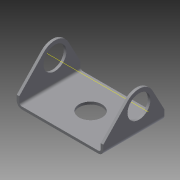
# Autodesk Inventor part: Bearing Mount 4 v1
Saved by Autodesk Inventor 2013 (Build 170138000, 138)
## iProperties
Created: 2013-01-18
Part Number: Bearing Mount 4 v1
Material: Generic
Document SubType Name: Sheet Metal
Designer: actoennies
Density: 1 g/cm^3
Flat Pattern Width: 7.62 cm
Flat Pattern Length: 19.8513 cm
Flat Pattern Area: 151.267 cm^2
Sheet Metal Rule: Default
Sheet Metal Width: 3.000 in
Sheet Metal Length: 7.815 in
Sheet Metal Area: 23.446 in^2
Mass: 35.0244 g
Surface Area: 244.107 cm^2
Volume: 35.0244 cm^3
Author: actoennies
Autodesk Inventor part; units mm, degrees
ref_plane "YZ Plane" through (0, 0, 0) normal (1, 0, 0) x (0, 1, 0)
ref_plane "XZ Plane" through (0, 0, 0) normal (0, 1, 0) x (-1, 0, 0)
ref_plane "XY Plane" through (0, 0, 0) normal (0, 0, 1) x (1, 0, 0)
sketch "Sketch1" plane through (0, 0, 0) normal (0, 1, 0) x (-1, 0, 0)
  line L0 (0, 0) -> (101.6, 0)
  line L1 (101.6, 0) -> (101.6, 76.2)
  line L2 (101.6, 76.2) -> (0, 76.2)
  line L3 (0, 76.2) -> (0, 0)
  dimension "d0" = 101.6
  dimension "d2" = 76.2
  measures "d0" distance of L1.end L2.end
  measures "d2" distance of L0.end L1.end
extrude "Plate1" add sketch "Sketch1" along normal blind 3.175
sketch "Sketch2" plane through (-101.6, 3.175, 76.2) normal (-1, 0, 0) x (0, -1, 0)
  line L0 (0, -76.2) -> (0, 0)
  line L1 (0, 0) -> (-47.625, 0)
  line L2 (-47.625, 0) -> (-47.625, -76.2)
  line L3 (-47.625, -76.2) -> (0, -76.2)
  constraints: 6 end point, 1 horizontal, 1 perpendicular, 1 vertical
edge flange "Flange1" height 50.8 angle 90 thickness 3.175 bend radius 3.175 thickness toward (-1, 0, 0) relief straight relief width 3.175 relief depth 1.5875 edges at (-101.6, 3.175, 38.1) wall of the first edge with corners at (-101.6, 3.175, 0) (-101.6, 3.175, 76.2) (-101.6, 50.8, 76.2) (-101.6, 50.8, 0)
bend "Bend1"
corner "Corner1"
sketch "Sketch3" plane through (0, 3.175, 0) normal (1, 0, 0) x (0, 1, 0)
  line L0 (0, 76.2) -> (0, 0)
  line L1 (0, 0) -> (47.625, 0)
  line L2 (47.625, 0) -> (47.625, 76.2)
  line L3 (47.625, 76.2) -> (0, 76.2)
  constraints: 6 end point, 1 horizontal, 1 perpendicular, 1 vertical
edge flange "Flange2" height 50.8 angle 90 thickness 3.175 bend radius 3.175 thickness toward (1, 0, 0) relief straight relief width 3.175 relief depth 1.5875 edges at (0, 3.175, 38.1) wall of the first edge with corners at (0, 3.175, 76.2) (0, 3.175, 0) (0, 50.8, 0) (0, 50.8, 76.2)
bend "Bend2"
corner "Corner2"
sketch "Sketch4" plane through (-101.6, 50.8, 76.2) normal (1, 0, 0) x (0, 0, -1)
  line L0 (76.2, 0) -> (0, 0) projected
  circle A0 centre (44.45, -19.05) radius 14.2875
  point P0 (76.2, -50.8)
  dimension "d24" = 28.575
  dimension "d25" = 19.05
  constraints: 1 centre point
  measures "d24" diameter of A0
  measures "d25" distance from line of L0 A0.centre
extrude "Cut1" cut sketch "Sketch4" against normal mid plane 5080
sketch "Sketch5" plane through (3.175, 50.8, 76.2) normal (1, 0, 0) x (0, 0, -1)
  circle A0 centre (44.45, -19.05) radius 14.2875 projected
  line L0 (0, -44.45) -> (76.2, -44.45) projected
  line L1 (76.2, 0) -> (76.2, -44.45) projected
  line L2 (0, 0) -> (76.2, 0) projected
  line L3 (0, -44.45) -> (0, 0) projected
  arc A1 (61.2588, -10.0853) -> (30.6552, -5.9121) centre (44.45, -19.05) ccw
  line L4 (0, -38.1) -> (30.6552, -5.9121)
  line L5 (61.2588, -10.0853) -> (76.2, -38.1)
  point P0 (76.2, -50.8)
  dimension "d28" = 6.35
  dimension "d29" = 6.35
  constraints: 4 end point, 2 point on circle, 2 point on line, 2 tangent, 1 centre point, 1 coincident, 1 other
  measures "d28" distance from line of L0 L4.start
  measures "d29" distance of L0.end L5.end
extrude "Cut2" cut sketch "Sketch5" against normal blind 508 contours L3 L2 A1 L4 | L5 A1 L2 L1
sketch "Sketch6" plane through (0, 3.175, 0) normal (0, 1, 0) x (1, 0, 0)
  circle A0 centre (-50.8, -38.1) radius 14.2875
  line L0 (-3.175, -76.2) -> (-3.175, 0) projected
  line L1 (-3.175, -76.2) -> (-98.425, -76.2) projected
  point P0 (0, 0)
  dimension "d32" = 28.575
  dimension "d35" = 38.1
  dimension "d36" = 47.625
  constraints: 1 centre point
  measures "d32" diameter of A0
  measures "d35" distance from line of L1 A0.centre
  measures "d36" distance from line of L0 A0.centre
extrude "Cut3" cut sketch "Sketch6" against normal blind 3.175
equation "\"d33\" = Thickness"
equation "\"d4\" = BendReliefWidth"
equation "\"d5\" = BendReliefDepth"
equation "\"d6\" = MinimumRemnant"
equation "\"d7\" = BendRadius"
equation "\"d10\" = BendRadius"
equation "\"d11\" = CornerReliefSize"
equation "\"d12\" = GapSize"
equation "\"d13\" = JacobiRadiusSize"
equation "\"d14\" = BendReliefWidth"
equation "\"d15\" = BendReliefDepth"
equation "\"d16\" = MinimumRemnant"
equation "\"d17\" = BendRadius"
equation "\"d20\" = BendRadius"
equation "\"d21\" = CornerReliefSize"
equation "\"d22\" = GapSize"
equation "\"d23\" = JacobiRadiusSize"
equation "\"BendRadius\" = Thickness"
equation "\"BendReliefWidth\" = Thickness"
equation "\"BendReliefDepth\" = 0.5 * Thickness"
equation "\"CornerReliefSize\" = 4 * Thickness"
equation "\"MinimumRemnant\" = 2 * Thickness"
equation "\"TransitionRadius\" = BendRadius"
equation "\"JacobiRadiusSize\" = BendRadius"
equation "\"GapSize\" = Thickness"
equation "\"d3\" = BendRadius"
equation "\"Thickness\" = 3.175"
body "Solid1"
